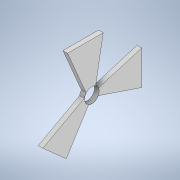
# Autodesk Inventor part: fan blade
Saved by Autodesk Inventor 2021 (Build 250183000, 183)
## iProperties
Created: 2021-07-18
Part Number: fan blade
Material: Generic
Document SubType Name: Modeling
Designer: HP
Density: 1 g/cm^3
Appearance: Default
Author: HP
Autodesk Inventor part; units mm, degrees
ref_plane "YZ Plane" through (0, 0, 0) normal (1, 0, 0) x (0, 1, 0)
ref_plane "XZ Plane" through (0, 0, 0) normal (0, 1, 0) x (-1, 0, 0)
ref_plane "XY Plane" through (0, 0, 0) normal (0, 0, 1) x (1, 0, 0)
sketch "Sketch1" plane through (0, 0, 0) normal (1, 0, 0) x (0, 1, 0)
  circle A0 centre (0, 0) radius 129
  circle A1 centre (0, 0) radius 125.5
  dimension "d0" = 258
  dimension "d1" = 251
  constraints: 2 centre point, 2 coincident
  measures "d0" diameter of A0
  measures "d1" diameter of A1
extrude "Extrusion1" add sketch "Sketch1" along normal blind 80
sketch "Sketch2" plane through (80, 0, 0) normal (1, 0, 0) x (0, 0, -1)
  line L0 (-101.4747, 92.723) -> (-414.8501, 828.7908)
  line L1 (-414.8501, 828.7908) -> (195.4959, 828.7908)
  line L2 (195.4959, 828.7908) -> (66.4648, 110.5596)
  circle A0 centre (0, 0) radius 129 projected
  line L3 (-101.4747, 92.723) -> (-97.8081, 84.1106)
  line L4 (118.8614, 50.1294) -> (856.9556, 272.0827)
  line L5 (856.9556, 272.0827) -> (856.9556, -315.7415)
  line L6 (856.9556, -315.7415) -> (112.0393, -63.9391)
  line L7 (-127.8547, 17.1518) -> (-838.6795, -370.3737)
  line L8 (-838.6795, -370.3737) -> (-437.3695, -726.566)
  line L9 (-437.3695, -726.566) -> (-54.85, -116.7582)
  dimension "d4" = 800
  constraints: 20 end point, 6 point on circle, 1 horizontal, 1 perpendicular, 1 point on line
  measures "d4" distance of L0.start L0.end
extrude "Extrusion2" add sketch "Sketch2" against normal blind 80 contours L0 L1 L2 A0 L3 | A0 L9 L8 L7 | L4 L5 L6 A0
body "Solid1"
